Autodesk Fusion 360 part; units mm, degrees
(part 4 of 4)
sketch "Sketch12" plane through (0, 0, 1.5) normal (0, 0, 1) x (-1, 0, 0)
  ellipse E0 centre (-19.3725, -71.5578) end of major axis (-15.5088, -72.5931) minor radius 1 (-19.6313, -72.5237) -> (-19.1137, -70.5919) ccw
  line L0 (-19.6313, -72.5237) -> (-28.477, -70.1535)
  ellipse E1 centre (-28.2182, -69.1876) end of major axis (-24.3375, -70.2275) minor radius 1 (-32.1062, -68.2428) -> (-28.477, -70.1535) ccw
  line L1 (-32.1062, -68.2428) -> (-32.0577, -68.0619)
  ellipse E2 centre (-28.2182, -69.1876) end of major axis (-24.3375, -70.2275) minor radius 1 (-27.9594, -68.2217) -> (-32.0577, -68.0619) ccw
  line L2 (-27.9594, -68.2217) -> (-19.1137, -70.5919)
  ellipse E3 centre (-74.6275, -71.5578) end of major axis (-70.7638, -70.5225) minor radius 1 (-74.8863, -70.5919) -> (-74.3687, -72.5237) ccw
  line L3 (-74.8863, -70.5919) -> (-66.0406, -68.2217)
  ellipse E4 centre (-65.7818, -69.1876) end of major axis (-61.9181, -68.1523) minor radius 1 (-65.523, -70.1535) -> (-66.0406, -68.2217) ccw
  line L4 (-65.523, -70.1535) -> (-74.3687, -72.5237)
  ellipse E5 centre (-19.2141, -80.8402) end of major axis (-15.75, -82.8402) minor radius 1 (-19.7141, -81.7063) -> (-18.7141, -79.9742) ccw
  line L5 (-19.7141, -81.7063) -> (-38.5359, -70.8395)
  ellipse E6 centre (-38.0359, -69.9735) end of major axis (-34.5718, -71.9735) minor radius 1 (-37.5359, -69.1074) -> (-38.5359, -70.8395) ccw
  line L6 (-37.5359, -69.1074) -> (-18.7141, -79.9742)
  ellipse E7 centre (-74.7859, -80.8402) end of major axis (-71.3218, -78.8402) minor radius 1 (-75.2859, -79.9742) -> (-74.2859, -81.7063) ccw
  line L7 (-75.2859, -79.9742) -> (-56.4641, -69.1074)
  ellipse E8 centre (-55.9641, -69.9735) end of major axis (-52.5, -67.9735) minor radius 1 (-55.4641, -70.8395) -> (-56.4641, -69.1074) ccw
  line L8 (-55.4641, -70.8395) -> (-74.2859, -81.7063)
  ellipse E9 centre (-56, -51.25) end of major axis (-52, -51.25) minor radius 1 (-56, -52.25) -> (-56, -50.25) ccw
  line L9 (-56, -52.25) -> (-74.75, -52.25)
  ellipse E10 centre (-74.75, -51.25) end of major axis (-70.75, -51.25) minor radius 1 (-74.75, -50.25) -> (-74.75, -52.25) ccw
  line L10 (-74.75, -50.25) -> (-56, -50.25)
  ellipse E11 centre (-74.75, -23.25) end of major axis (-70.75, -23.25) minor radius 1 (-74.75, -22.25) -> (-74.75, -24.25) ccw
  line L11 (-74.75, -22.25) -> (-56, -22.25)
  ellipse E12 centre (-56, -23.25) end of major axis (-52, -23.25) minor radius 1 (-56, -24.25) -> (-56, -22.25) ccw
  line L12 (-56, -24.25) -> (-74.75, -24.25)
  ellipse E13 centre (-38, -30.25) end of major axis (-34, -30.25) minor radius 1 (-38, -29.25) -> (-38, -31.25) ccw
  line L13 (-38, -29.25) -> (-19.25, -29.25)
  ellipse E14 centre (-19.25, -30.25) end of major axis (-15.25, -30.25) minor radius 1 (-19.25, -31.25) -> (-19.25, -29.25) ccw
  line L14 (-19.25, -31.25) -> (-38, -31.25)
  ellipse E15 centre (-38, -58.25) end of major axis (-34, -58.25) minor radius 1 (-38, -57.25) -> (-38, -59.25) ccw
  line L15 (-38, -57.25) -> (-19.25, -57.25)
  ellipse E16 centre (-19.25, -58.25) end of major axis (-15.25, -58.25) minor radius 1 (-19.25, -59.25) -> (-19.25, -57.25) ccw
  line L16 (-19.25, -59.25) -> (-38, -59.25)
  ellipse E17 centre (-19.25, -51.25) end of major axis (-15.25, -51.25) minor radius 1 (-19.25, -52.25) -> (-19.25, -50.25) ccw
  line L17 (-19.25, -52.25) -> (-38, -52.25)
  ellipse E18 centre (-38, -51.25) end of major axis (-34, -51.25) minor radius 1 (-38, -50.25) -> (-38, -52.25) ccw
  line L18 (-38, -50.25) -> (-19.25, -50.25)
  ellipse E19 centre (-19.25, -23.25) end of major axis (-15.25, -23.25) minor radius 1 (-19.25, -24.25) -> (-19.25, -22.25) ccw
  line L19 (-19.25, -24.25) -> (-38, -24.25)
  ellipse E20 centre (-38, -23.25) end of major axis (-34, -23.25) minor radius 1 (-38, -22.25) -> (-38, -24.25) ccw
  line L20 (-38, -22.25) -> (-19.25, -22.25)
  ellipse E21 centre (-74.75, -30.25) end of major axis (-70.75, -30.25) minor radius 1 (-74.75, -29.25) -> (-74.75, -31.25) ccw
  line L21 (-74.75, -29.25) -> (-56, -29.25)
  ellipse E22 centre (-56, -30.25) end of major axis (-52, -30.25) minor radius 1 (-56, -31.25) -> (-56, -29.25) ccw
  line L22 (-56, -31.25) -> (-74.75, -31.25)
  ellipse E23 centre (-74.75, -58.25) end of major axis (-70.75, -58.25) minor radius 1 (-74.75, -57.25) -> (-74.75, -59.25) ccw
  line L23 (-74.75, -57.25) -> (-56, -57.25)
  ellipse E24 centre (-56, -58.25) end of major axis (-52, -58.25) minor radius 1 (-56, -59.25) -> (-56, -57.25) ccw
  line L24 (-56, -59.25) -> (-74.75, -59.25)
  ellipse E25 centre (-74.75, -44.25) end of major axis (-70.75, -44.25) minor radius 1 (-74.75, -43.25) -> (-74.75, -45.25) ccw
  line L25 (-74.75, -43.25) -> (-56, -43.25)
  ellipse E26 centre (-56, -44.25) end of major axis (-52, -44.25) minor radius 1 (-56, -45.25) -> (-56, -43.25) ccw
  line L26 (-56, -45.25) -> (-74.75, -45.25)
  ellipse E27 centre (-74.75, -16.25) end of major axis (-70.75, -16.25) minor radius 1 (-74.75, -15.25) -> (-74.75, -17.25) ccw
  line L27 (-74.75, -15.25) -> (-56, -15.25)
  ellipse E28 centre (-56, -16.25) end of major axis (-52, -16.25) minor radius 1 (-56, -17.25) -> (-56, -15.25) ccw
  line L28 (-56, -17.25) -> (-74.75, -17.25)
  ellipse E29 centre (-19.25, -37.25) end of major axis (-15.25, -37.25) minor radius 1 (-19.25, -38.25) -> (-19.25, -36.25) ccw
  line L29 (-19.25, -38.25) -> (-38, -38.25)
  ellipse E30 centre (-38, -37.25) end of major axis (-34, -37.25) minor radius 1 (-38, -36.25) -> (-38, -38.25) ccw
  line L30 (-38, -36.25) -> (-19.25, -36.25)
  ellipse E31 centre (-19.25, -65.25) end of major axis (-15.25, -65.25) minor radius 1 (-19.25, -66.25) -> (-19.25, -64.25) ccw
  line L31 (-19.25, -66.25) -> (-38, -66.25)
  ellipse E32 centre (-38, -65.25) end of major axis (-34, -65.25) minor radius 1 (-38, -64.25) -> (-38, -66.25) ccw
  line L32 (-38, -64.25) -> (-19.25, -64.25)
  ellipse E33 centre (-38, -44.25) end of major axis (-34, -44.25) minor radius 1 (-38, -43.25) -> (-38, -45.25) ccw
  line L33 (-38, -43.25) -> (-19.25, -43.25)
  ellipse E34 centre (-19.25, -44.25) end of major axis (-15.25, -44.25) minor radius 1 (-19.25, -45.25) -> (-19.25, -43.25) ccw
  line L34 (-19.25, -45.25) -> (-38, -45.25)
  ellipse E35 centre (-38, -16.25) end of major axis (-34, -16.25) minor radius 1 (-38, -15.25) -> (-38, -17.25) ccw
  line L35 (-38, -15.25) -> (-19.25, -15.25)
  ellipse E36 centre (-19.25, -16.25) end of major axis (-15.25, -16.25) minor radius 1 (-19.25, -17.25) -> (-19.25, -15.25) ccw
  line L36 (-19.25, -17.25) -> (-38, -17.25)
  line L37 (-74.75, -36.25) -> (-56, -36.25)
  ellipse E37 centre (-56, -37.25) end of major axis (-52, -37.25) minor radius 1 (-56, -38.25) -> (-56, -36.25) ccw
  line L38 (-56, -38.25) -> (-74.75, -38.25)
  ellipse E38 centre (-74.75, -37.25) end of major axis (-70.75, -37.25) minor radius 1 (-74.75, -36.25) -> (-74.75, -38.25) ccw
  ellipse E39 centre (-74.75, -65.25) end of major axis (-70.75, -65.25) minor radius 1 (-74.75, -64.25) -> (-74.75, -66.25) ccw
  line L39 (-74.75, -64.25) -> (-56, -64.25)
  ellipse E40 centre (-56, -65.25) end of major axis (-52, -65.25) minor radius 1 (-56, -66.25) -> (-56, -64.25) ccw
  line L40 (-56, -66.25) -> (-74.75, -66.25)
  line L41 (-34.7574, -85.9106) -> (-28.1106, -92.5574)
  ellipse E41 centre (-28.8177, -93.2645) end of major axis (-25.9892, -96.0929) minor radius 1 (-29.5248, -93.9716) -> (-28.1106, -92.5574) ccw
  line L42 (-29.5248, -93.9716) -> (-36.1716, -87.3248)
  ellipse E42 centre (-35.4645, -86.6177) end of major axis (-32.636, -89.4461) minor radius 1 (-34.7574, -85.9106) -> (-36.1716, -87.3248) ccw
  ellipse E43 centre (-73.5355, -93.2645) end of major axis (-70.7071, -90.436) minor radius 1 (-74.2426, -92.5574) -> (-72.8284, -93.9716) ccw
  line L43 (-74.2426, -92.5574) -> (-56.8095, -75.1242)
  ellipse E44 centre (-56.1024, -75.8313) end of major axis (-53.2739, -73.0029) minor radius 1 (-55.3953, -76.5384) -> (-56.8095, -75.1242) ccw
  line L44 (-55.3953, -76.5384) -> (-72.8284, -93.9716)
  ellipse E45 centre (-38.4645, -75.7892) end of major axis (-35.636, -78.6177) minor radius 1 (-37.7574, -75.0821) -> (-39.1716, -76.4963) ccw
  line L45 (-37.7574, -75.0821) -> (-20.2821, -92.5574)
  ellipse E46 centre (-20.9892, -93.2645) end of major axis (-18.1608, -96.0929) minor radius 1 (-21.6963, -93.9716) -> (-20.2821, -92.5574) ccw
  line L46 (-21.6963, -93.9716) -> (-39.1716, -76.4963)
  ellipse E47 centre (-58.5355, -93.9213) end of major axis (-55.7071, -91.0929) minor radius 1 (-57.5048, -94.2952) -> (-58.9094, -92.8906) ccw
  ellipse E48 centre (-57.8787, -93.2645) end of major axis (-55.0503, -90.436) minor radius 1 (-58.9094, -92.8906) -> (-57.5048, -94.2952) ccw
  ellipse E49 centre (-65.7071, -93.2645) end of major axis (-62.8787, -90.436) minor radius 1 (-66.4142, -92.5574) -> (-65, -93.9716) ccw
  line L47 (-66.4142, -92.5574) -> (-59.2426, -85.3858)
  ellipse E50 centre (-58.5355, -86.0929) end of major axis (-55.7071, -83.2645) minor radius 1 (-57.8284, -86.8) -> (-59.2426, -85.3858) ccw
  line L48 (-57.8284, -86.8) -> (-65, -93.9716)
  ellipse E51 centre (-35.6289, -93.7569) end of major axis (-32.8005, -96.5853) minor radius 1 (-35.1707, -92.8062) -> (-36.5796, -94.2151) ccw
  ellipse E52 centre (-36.1213, -93.2645) end of major axis (-33.2929, -96.0929) minor radius 1 (-36.5796, -94.2151) -> (-35.1707, -92.8062) ccw
  line L49 (-93.75, -111.8) -> (-0.25, -111.8)
  line L50 (-0.25, -111.8) -> (-0.25, -0.25)
  line L51 (-0.25, -0.25) -> (-93.75, -0.25)
  line L52 (-93.75, -0.25) -> (-93.75, -111.8)
  circle A0 centre (-3.5, -95.55) radius 2
  circle A1 centre (-90.5, -95.55) radius 2
  line L53 (-42.5, -83.8) -> (-42.5, -96.8)
  line L54 (-42.5, -96.8) -> (-51.5, -96.8)
  line L55 (-51.5, -96.8) -> (-51.5, -83.8)
  line L56 (-51.5, -83.8) -> (-42.5, -83.8)
  line L57 (-42, -100.3) -> (-42, -110.3)
  line L58 (-42, -110.3) -> (-43.9689, -110.3)
  line L59 (-43.9689, -110.3) -> (-43.9689, -103.55)
  line L60 (-43.9689, -103.55) -> (-47, -101.8)
  line L61 (-47, -101.8) -> (-50.0311, -103.55)
  line L62 (-50.0311, -103.55) -> (-50.0311, -110.3)
  line L63 (-50.0311, -110.3) -> (-52, -110.3)
  line L64 (-52, -110.3) -> (-52, -100.3)
  line L65 (-52, -100.3) -> (-55, -100.3)
  line L66 (-55, -100.3) -> (-55, -80.3)
  line L67 (-55, -80.3) -> (-52, -80.3)
  line L68 (-52, -80.3) -> (-52, -81.8)
  line L69 (-52, -81.8) -> (-53.5, -81.8)
  line L70 (-53.5, -81.8) -> (-53.5, -98.8)
  line L71 (-53.5, -98.8) -> (-40.5, -98.8)
  line L72 (-40.5, -98.8) -> (-40.5, -81.8)
  line L73 (-40.5, -81.8) -> (-42, -81.8)
  line L74 (-42, -81.8) -> (-42, -80.3)
  line L75 (-42, -80.3) -> (-39, -80.3)
  line L76 (-39, -80.3) -> (-39, -100.3)
  line L77 (-39, -100.3) -> (-42, -100.3)
  line L78 (-93.75, -0.25) -> (-88.75, -0.25)
  line L79 (-88.75, -0.25) -> (-88.75, -5.25)
  line L80 (-88.75, -5.25) -> (-93.75, -5.25)
  line L81 (-93.75, -5.25) -> (-93.75, -0.25)
  line L82 (-0.25, -0.25) -> (-6.75, -0.25)
  line L83 (-6.75, -0.25) -> (-6.75, -6.75)
  line L84 (-6.75, -6.75) -> (-0.25, -6.75)
  line L85 (-0.25, -6.75) -> (-0.25, -0.25)
  circle A2 centre (-6.75, -6.75) radius 2
  circle A3 centre (-88.75, -5.25) radius 2
  dimension "d261" = 5
  dimension "d262" = 5
  dimension "d263" = 6.5
  dimension "d264" = 6.5
  dimension "d265" = 4
  dimension "d266" = 4
  constraint horizontal L78
  constraint vertical L79
  constraint horizontal L80
  constraint vertical L81
  constraint coincident L51.end L52.start
  constraint horizontal L82
  constraint vertical L83
  constraint horizontal L84
  constraint vertical L85
  constraint coincident L50.end L51.start
  constraint coincident L83.end L84.start
  constraint coincident L79.end L80.start
  measures "d261" distance of L51.end L78.end
  measures "d262" distance of L51.end L80.end
  measures "d263" distance of L50.end L82.end
  measures "d264" distance of L50.end L84.end
  measures "d265" diameter of A2
  measures "d266" diameter of A3
extrude "Extrude16" cut sketch "Sketch12" against normal blind 1.5 contours L79 L80 A3 | L79 L80 A3 | L83 L84 A2 | L83 L84 A2
